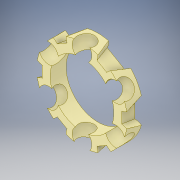
# Autodesk Inventor part: Bearings - Retainer
Saved by Autodesk Inventor 2019 (Build 230136000, 136)
## iProperties
Created: 2020-12-03
Part Number: Bearings - Retainer
Material: Nylon 6
Document SubType Name: Modeling
Designer: Anass Hamdi
Density: 1.12 g/cm^3
Appearance: Nylon 6
Author: Anass Hamdi
Autodesk Inventor part; units mm, degrees
ref_plane "YZ Plane" through (0, 0, 0) normal (1, 0, 0) x (0, 1, 0)
ref_plane "XZ Plane" through (0, 0, 0) normal (0, 1, 0) x (-1, 0, 0)
sketch "Sketch1" plane through (0, 0, 0) normal (0, 0, 1) x (1, 0, 0)
  circle A0 centre (0, 0) radius 6
  circle A1 centre (0, 0) radius 8.5
  dimension "d0" = 12
  dimension "d1" = 17
  constraints: 2 centre point, 2 coincident
  measures "d0" diameter of A0
  measures "d1" diameter of A1
extrude "Extrusion1" add sketch "Sketch1" along normal mid plane 3
sketch "Sketch8" plane through (0, 0, -1.5) normal (0, 0, -1) x (-1, 0, 0)
  arc A0 (-8.1494, 2.4161) -> (-6.9282, 2) centre (-6.9282, 4) ccw
  arc A1 (-6.9282, -2) -> (-8.1494, -2.4161) centre (-6.9282, -4) ccw
  line L0 (-6.9282, 2) -> (-6.9282, -2)
  line L1 (-8.1494, 2.4161) -> (-9.6249, 2.4161)
  line L2 (-8.1494, -2.4161) -> (-9.6249, -2.4161)
  line L3 (-9.6249, -2.4161) -> (-9.6249, 2.4161)
  point P0 (0, 0)
  dimension "d66" = 2
  constraints: 8 end point, 4 point on circle, 2 centre point, 2 coincident, 2 horizontal, 1 perpendicular, 1 vertical
  measures "d66" radius of A0
sketch "Sketch9" plane through (0, 0, 1.5) normal (0, 0, 1) x (1, 0, 0)
  arc A0 (8.3874, -1.3788) -> (7.4675, -1.0489) centre (6.9282, -4) ccw
  arc A1 (7.4675, 1.0489) -> (8.3874, 1.3788) centre (6.9282, 4) ccw
  line L0 (7.4675, -1.0489) -> (7.4675, 1.0489)
  line L1 (9.6249, -1.3788) -> (9.6249, 1.3788)
  line L2 (8.3874, -1.3788) -> (9.6249, -1.3788)
  line L3 (8.3874, 1.3788) -> (9.6249, 1.3788)
  point P0 (0, 0)
  dimension "d67" = 6
  dimension "d68" = 6
  constraints: 8 end point, 4 point on circle, 2 centre point, 2 coincident, 1 horizontal, 1 parallel, 1 vertical
  measures "d67" diameter of A0
  measures "d68" diameter of A1
loft "Loft3" cut profiles "Sketch8", "Sketch9"
pattern_circular "Circular Pattern6" count 6 over 360 about axis through (0, 0, 0) along (0, 0, 1) of "Loft3"
ref_plane "Work Plane1" through (0, 0, 0.75) normal (0, 0, 1) x (1, 0, 0)
sketch "Sketch10" plane through (0, 0, 0.75) normal (0, 0, 1) x (1, 0, 0)
  line L0 (0, -7.75) -> (0, -5.25) construction
  arc A0 (0, -5.25) -> (0, -9.25) centre (0, -7.25) ccw
  line L1 (0, -9.25) -> (0, -5.25)
  point P0 (0, 0)
  point P1 (0, 0)
  dimension "d78" = 2
  constraints: 4 end point, 2 coincident, 2 point on circle, 2 vertical, 1 centre point, 1 point on line, 1 other
  measures "d78" radius of A0
revolve "Revolution7" cut sketch "Sketch10" angle 360 about axis through (0, -9.25, 0.75) along (0, 1, 0)
pattern_circular "Circular Pattern7" count 6 over 360 about axis through (0, 0, 0) along (0, 0, 1) of "Revolution7"
equation "\"d22\" = d21"
equation "\"d21\" = 6"
body "Solid1"
